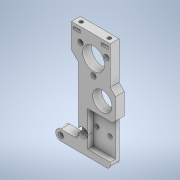
# Autodesk Inventor part: PartA_3D
Saved by Autodesk Inventor 2020.2 (Build 242310000, 310)
## iProperties
Created: 2020-12-02
Part Number: PartA_3D
Material: Generic
Document SubType Name: Modeling
Designer: Acer
Density: 1 g/cm^3
Appearance: Default
Author: Acer
Autodesk Inventor part; units mm, degrees
ref_plane "YZ Plane" through (0, 0, 0) normal (1, 0, 0) x (0, 1, 0)
ref_plane "XZ Plane" through (0, 0, 0) normal (0, 1, 0) x (-1, 0, 0)
ref_plane "XY Plane" through (0, 0, 0) normal (0, 0, 1) x (1, 0, 0)
sketch "Sketch1" plane through (0, 0, 0) normal (0, 0, 1) x (1, 0, 0)
  circle A0 centre (0, 0) radius 1.5
  circle A1 centre (0, 0) radius 3
  line L0 (0, 3) -> (28, 3)
  line L1 (28, 3) -> (28, -3)
  line L2 (28, -3) -> (0, -3)
  line L3 (0, -3) -> (0, 3)
  line L4 (28, 3) -> (10, 3)
  line L5 (10, 3) -> (10, 59)
  line L6 (10, 59) -> (28, 59)
  line L7 (28, 59) -> (28, 3)
  circle A2 centre (23.5, 28.5) radius 5.5
  circle A3 centre (18.553, 47) radius 6.25
  line L8 (23.5, 28.5) -> (18.553, 47) construction
  line L9 (23.5, 28.5) -> (10, 28.5) construction
  circle A4 centre (18.553, 38.5) radius 0.8
  circle A5 centre (25.9142, 51.25) radius 0.8
  circle A6 centre (11.1918, 51.25) radius 0.8
  line L10 (10, 59) -> (6, 59)
  line L11 (6, 59) -> (6, 45)
  line L12 (6, 45) -> (10, 45)
  line L13 (10, 45) -> (10, 59)
  line L14 (6, 45) -> (10, 41)
  line L15 (6, 45) -> (11.6569, 45) construction
  line L16 (28, 34.5) -> (31, 34.5)
  line L17 (31, 34.5) -> (31, 22.5)
  line L18 (31, 22.5) -> (28, 22.5)
  line L19 (28, 22.5) -> (28, 34.5)
  line L20 (31, 34.5) -> (28, 37.5)
  line L21 (31, 34.5) -> (35.2426, 34.5) construction
  line L22 (31, 22.5) -> (28, 19.5)
  line L23 (31, 22.5) -> (35.2426, 22.5) construction
  circle A7 centre (12.5, 7.5) radius 1.5
  circle A8 centre (17.5, 11.5) radius 1.25
  circle A9 centre (25, 10.5) radius 1.25
  line L24 (18.553, 47) -> (6, 47) construction
  line L25 (18.553, 38.5) -> (18.553, 47) construction
  dimension "d0" = 3
  dimension "d1" = 6
  dimension "d2" = 28
  dimension "d3" = 6
  dimension "d4" = 0
  dimension "d5" = 3
  dimension "d6" = 18
  dimension "d7" = 56
  dimension "d8" = 11
  dimension "d9" = 4.5
  dimension "d10" = 25.5
  dimension "d11" = 12.5
  dimension "d12" = 19.15
  dimension "d14" = 1.6
  dimension "d17" = 12
  dimension "d20" = 360
  dimension "d22" = 4
  dimension "d23" = 14
  dimension "d24" = 45
  dimension "d25" = 3
  dimension "d26" = 12
  dimension "d27" = 6
  dimension "d28" = 135
  dimension "d29" = 135
  dimension "d32" = 3
  dimension "d33" = 10.5
  dimension "d34" = 2.5
  dimension "d35" = 2.5
  dimension "d36" = 14.5
  dimension "d37" = 7.5
  dimension "d38" = 2.5
  dimension "d39" = 15
  dimension "d40" = 13.5
  dimension "d60" = 8.5
  dimension "d61" = 270
  constraints: 52 end point, 10 centre point, 8 horizontal, 8 parallel, 6 point on line, 5 perpendicular, 3 equal length, 2 coincident, 7 other
  measures "d0" diameter of A0
  measures "d1" diameter of A1
  measures "d2" distance of L1.end L2.end
  measures "d3" distance of L0.end L1.end
  measures "d4" distance from line of point (0, 0) L3
  measures "d5" distance from line of L0 point (0, 0)
  measures "d6" distance of L5.end L6.end
  measures "d7" distance of L4.end L5.end
  measures "d8" diameter of A2
  measures "d9" distance from line of L7 L8.start
  measures "d10" distance from line of L8.start L0
  measures "d11" diameter of A3
  measures "d12" distance of L8.start L8.end
  measures "d14" diameter of A4
  measures "d17" distance from line of L6 L8.end
  measures "d22" distance of L12.end L11.end
  measures "d23" distance of L11.end L10.end
  measures "d24" angle of L14 L15
  measures "d25" distance of L17.end L18.end
  measures "d26" distance of L16.end L17.end
  measures "d27" distance from line of L16 L8.start
  measures "d28" angle of L21 L20
  measures "d29" angle of L22 L23
  measures "d32" diameter of A7
  measures "d33" distance from line of L2 A7.centre
  measures "d34" distance from line of L5 A7.centre
  measures "d35" diameter of A8
  measures "d36" distance from line of A8.centre L2
  measures "d37" distance from line of L5 A8.centre
  measures "d38" diameter of A9
  measures "d39" distance from line of A9.centre L5
  measures "d40" distance from line of L2 A9.centre
  measures "d60" distance of L25.start L8.end
extrude "Extrusion1" add sketch "Sketch1" along normal blind 5 contours A0 L3 A1 | A0 L3 A1 | L0 L1 L2 A1 | L5 L6 L7 A2 L0 | L14 L12 L5 | L7 L18 L22 | L12 L11 L10 L5 | L7 A2 L16 L17 L18 | L16 L7 L20
fillet "Fillet1" radius 2 1 edges at (28, -3, 2.5)
fillet "Fillet2" radius 2 1 edges at (10, 3, 2.5)
sketch "Sketch2" plane through (0, 0, 5) normal (0, 0, 1) x (1, 0, 0)
  line L0 (28, -1) -> (28, 19.5) projected
  line L1 (0, -3) -> (26, -3) projected
  line L2 (28, -1) -> (28, 19.5) projected
  line L3 (28, 20.75) -> (15.25, 20.75)
  line L4 (15.25, 20.75) -> (15.25, 0.75)
  line L5 (15.25, 0.75) -> (28, 0.75)
  line L6 (28, 0.75) -> (28, 20.75)
  line L7 (28, 19.5) -> (31, 22.5) projected
  line L8 (28, 20.75) -> (29.25, 20.75)
  line L9 (28, 19.5) -> (31, 22.5) projected
  point P0 (0, 0)
  point P1 (28, 19.5)
  point P2 (28, 19.5)
  dimension "d43" = 12.75
  dimension "d44" = 20
  dimension "d45" = 23.75
  constraints: 10 end point, 2 horizontal, 2 parallel, 2 point on line, 1 perpendicular
  measures "d43" distance of L5.end L4.end
  measures "d44" distance of L4.end L3.end
  measures "d45" distance between parallel lines of L1 L3
extrude "Extrusion2" cut sketch "Sketch2" against normal blind 3
sketch "Sketch3" plane through (6, 59, 0) normal (0, 1, 0) x (1, 0, 0)
  circle A0 centre (3, -2.5) radius 1
  line L0 (22, 0) -> (0, 0) projected
  line L1 (0, 0) -> (0, -5) projected
  line L2 (22, -5) -> (0, -5) projected
  line L3 (22, 0) -> (22, -5) projected
  circle A1 centre (19, -2.5) radius 1
  dimension "d48" = 2
  dimension "d49" = 2
  dimension "d50" = 2.5
  dimension "d51" = 2.5
  dimension "d52" = 3
  dimension "d53" = 3
  constraints: 2 centre point
  measures "d48" diameter of A0
  measures "d49" diameter of A1
  measures "d50" distance from line of L0 A0.centre
  measures "d51" distance from line of L0 A1.centre
  measures "d52" distance from line of A1.centre L3
  measures "d53" distance from line of L1 A0.centre
extrude "Extrusion3" cut sketch "Sketch3" against normal blind 6 contours A0 | A1
thread "Thread1" size "M2x0.4" class "6H" standard "ANSI Metric M Profile" length 7
thread "Thread2" size "M2x0.4" class "6H" standard "ANSI Metric M Profile" length 7
sketch "Sketch5" plane through (0, 0, 5) normal (0, 0, 1) x (1, 0, 0)
  circle A0 centre (18.553, 38.5) radius 0.8 projected
  circle A1 centre (11.1918, 51.25) radius 0.8 projected
  circle A2 centre (25.9142, 51.25) radius 0.8 projected
  circle A3 centre (18.553, 38.5) radius 1.5
  circle A4 centre (11.1918, 51.25) radius 1.5
  circle A5 centre (25.9142, 51.25) radius 1.5
  point P0 (0, 0)
  dimension "d62" = 3
  dimension "d63" = 3
  dimension "d64" = 3
  constraints: 3 centre point, 3 coincident
  measures "d62" diameter of A3
  measures "d63" diameter of A4
  measures "d64" diameter of A5
extrude "Extrusion4" cut sketch "Sketch5" against normal blind 3 contours A0 | A1 | A2 | A3 | A4 | A5
sketch "Sketch7" plane through (0, 0, 5) normal (0, 0, 1) x (1, 0, 0)
  circle A0 centre (12.5, 7.5) radius 1.5 projected
  circle A1 centre (12.5, 7.5) radius 2.75
  point P0 (0, 0)
  dimension "d67" = 5.5
  constraints: 1 centre point, 1 coincident
  measures "d67" diameter of A1
extrude "Extrusion5" cut sketch "Sketch7" against normal blind 2 contours A0 | A1
sketch "Sketch8" plane through (0, 0, 5) normal (0, 0, 1) x (1, 0, 0)
  line L0 (10, 59) -> (10, 53) projected
  line L1 (8, 59) -> (8, 53) projected
  circle A0 centre (25.9142, 51.25) radius 1.5 projected
  circle A1 centre (11.1918, 51.25) radius 1.5 projected
  circle A2 centre (18.553, 38.5) radius 1.5 projected
  circle A3 centre (23.5, 28.5) radius 5.5 projected
  circle A4 centre (18.553, 47) radius 6.25 projected
  arc A5 (15.25, 7.5) -> (10, 8.6456) centre (12.5, 7.5) ccw projected
  line L2 (15.25, 7.5) -> (15.25, 20.75) projected
  line L3 (15.25, 20.75) -> (29.25, 20.75) projected
  line L4 (29.25, 20.75) -> (31, 22.5) projected
  line L5 (31, 22.5) -> (31, 34.5) projected
  line L6 (31, 34.5) -> (28, 37.5) projected
  line L7 (28, 37.5) -> (28, 59) projected
  line L8 (28, 59) -> (6, 59) projected
  line L9 (6, 59) -> (6, 45) projected
  line L10 (6, 45) -> (10, 41) projected
  line L11 (10, 41) -> (10, 8.6456) projected
  line L12 (24, 59) -> (24, 53) projected
  line L13 (26, 59) -> (26, 53) projected
  line L14 (7, 55.7) -> (11, 55.7)
  line L15 (11, 55.7) -> (11, 57.3)
  line L16 (11, 57.3) -> (7, 57.3)
  line L17 (7, 57.3) -> (7, 55.7)
  line L18 (7, 55.7) -> (11, 57.3) construction
  line L19 (11, 55.7) -> (7, 57.3) construction
  line L20 (23, 57.3) -> (27, 57.3)
  line L21 (27, 57.3) -> (27, 55.7)
  line L22 (27, 55.7) -> (23, 55.7)
  line L23 (23, 55.7) -> (23, 57.3)
  line L24 (23, 57.3) -> (27, 55.7) construction
  line L25 (27, 57.3) -> (23, 55.7) construction
  point P0 (0, 0)
  point P1 (9, 56.5)
  point P2 (25, 56.5)
  dimension "d70" = 4
  dimension "d71" = 1.6
  dimension "d72" = 4
  dimension "d73" = 1.6
  dimension "d74" = 1
  dimension "d75" = 2.5
  dimension "d76" = 2.5
  dimension "d77" = 1
  constraints: 24 end point, 4 midpoint, 4 parallel, 2 horizontal, 2 perpendicular
  measures "d70" distance of L16.end L15.end
  measures "d71" distance of L15.end L14.end
  measures "d72" distance of L21.end L22.end
  measures "d73" distance of L20.end L21.end
  measures "d74" distance from line of point (9, 56.5) L0
  measures "d75" distance from line of L8 point (9, 56.5)
  measures "d76" distance from line of L8 point (25, 56.5)
  measures "d77" distance from line of point (25, 56.5) L13
extrude "Extrusion6" cut sketch "Sketch8" against normal up to surface (5 mm away) contours L16 L15 L14 L0 | L0 L14 L1 L16 | L1 L14 L17 L16 | L20 L13 L22 L12 | L12 L22 L23 L20 | L20 L21 L22 L13
body "Solid1"
